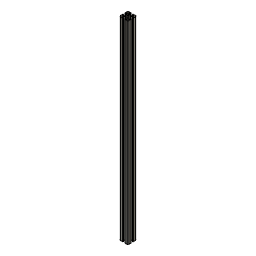
40mm X 40mm 3ft v2 (Autodesk Fusion 360 design; units mm, degrees)
Autodesk Fusion 360 part; units mm, degrees
sketch "Sketch1" plane through (0, 0, 0) normal (0, 0, 1) x (1, 0, 0)
  line L0 (4, 0) -> (14.435, 0)
  line L1 (40, 0) -> (40, 36)
  line L2 (36, 40) -> (0, 40)
  line L3 (0, 40) -> (0, 4)
  line L4 (0, 0) -> (0, 20)
  line L5 (0, 40) -> (20, 40)
  circle A0 centre (20, 20) radius 3.405
  line L6 (40, 40) -> (24.065, 40)
  line L7 (40, 40) -> (25.565, 40)
  line L8 (40, 40) -> (40, 25.565)
  line L9 (38.5, 24.065) -> (37.18, 24.065)
  line L10 (24.065, 38.5) -> (24.065, 37.18)
  line L11 (25.565, 35.68) -> (30.4344, 35.68)
  line L12 (35.68, 25.565) -> (35.68, 30.2904)
  line L13 (20, 20) -> (20, 40)
  line L14 (20, 20) -> (0, 20)
  line L15 (20, 20) -> (20, 0)
  line L16 (20, 20) -> (40, 20)
  line L17 (14.435, 35.68) -> (9.5498, 35.68)
  line L18 (15.935, 38.5) -> (15.935, 37.18)
  line L19 (4, 40) -> (14.435, 40)
  line L20 (0, 36) -> (0, 25.565)
  line L21 (1.5, 24.065) -> (2.8205, 24.065)
  line L22 (4.3205, 25.5645) -> (4.3219, 30.271)
  line L23 (25.565, 4.32) -> (1890698.4728, 3)
  line L24 (24.065, 1.5) -> (24.065, 2.82)
  line L25 (36, 0) -> (25.565, 0)
  line L26 (40, 4) -> (40, 14.435)
  line L27 (38.5, 15.935) -> (37.18, 15.935)
  line L28 (35.68, 14.435) -> (35.68, 9.7153)
  line L29 (14.435, 4.32) -> (9.7085, 4.32)
  line L30 (15.935, 1.5) -> (15.935, 2.82)
  line L31 (0, 0) -> (15.935, 0)
  line L32 (1.5, 15.935) -> (2.82, 15.935)
  line L33 (4.32, 14.435) -> (4.32, 9.5656)
  line L34 (0, 14.435) -> (0, 0)
  line L35 (0, 0) -> (15.935, 0)
  line L36 (5.9379, 30.9139) -> (12.3015, 24.1858)
  line L37 (8.8698, 34.1008) -> (15.0285, 27.5893)
  line L38 (30.9385, 5.9323) -> (24.4402, 12.1491)
  line L39 (33.9887, 8.9927) -> (27.7337, 14.9768)
  line L40 (5.903, 8.8892) -> (12.2663, 14.9767)
  line L41 (9.0615, 5.9323) -> (15.5598, 12.1491)
  line L42 (31.1111, 34.0973) -> (24.8873, 27.5855)
  line L43 (33.957, 30.8226) -> (27.7021, 24.2782)
  line L44 (27.425, 23.5872) -> (27.425, 15.6993)
  line L45 (16.2511, 12.4265) -> (23.7489, 12.4265)
  line L46 (12.575, 15.6993) -> (12.575, 23.4986)
  line L47 (15.7551, 27.2765) -> (24.1644, 27.2765)
  line L48 (35.68, 30.1316) -> (35.68, 30.2853)
  line L49 (34.0667, 30.9373) -> (34.0632, 30.9337)
  arc A1 (33.9887, 8.9927) -> (35.68, 9.7153) centre (34.68, 9.7153) ccw
  line L50 (35.68, 7.3747) -> (35.68, 9.7153)
  arc A2 (27.7021, 24.2782) -> (27.425, 23.5872) centre (28.425, 23.5872) ccw
  arc A3 (35.68, 30.2904) -> (34.0667, 30.9373) centre (34.7436, 30.2904) ccw
  arc A4 (5.9379, 30.9139) -> (4.3219, 30.271) centre (5.2579, 30.2707) ccw
  arc A5 (12.575, 23.4986) -> (12.3015, 24.1858) centre (11.575, 23.4986) ccw
  arc A6 (12.2663, 14.9767) -> (12.575, 15.6993) centre (11.575, 15.6993) ccw
  arc A7 (4.32, 9.5656) -> (5.903, 8.8892) centre (5.256, 9.5656) ccw
  arc A8 (9.0615, 5.9323) -> (9.7085, 4.32) centre (9.7085, 5.256) ccw
  arc A9 (30.2914, 4.32) -> (30.9385, 5.9323) centre (30.2914, 5.256) ccw
  arc A10 (24.4402, 12.1491) -> (23.7489, 12.4265) centre (23.7489, 11.4265) ccw
  arc A11 (16.2511, 12.4265) -> (15.5598, 12.1491) centre (16.2511, 11.4265) ccw
  arc A12 (27.425, 15.6993) -> (27.7337, 14.9768) centre (28.425, 15.6993) ccw
  arc A13 (24.1644, 27.2765) -> (24.8873, 27.5855) centre (24.1644, 28.2765) ccw
  arc A14 (15.0285, 27.5893) -> (15.7551, 27.2765) centre (15.7551, 28.2765) ccw
  arc A15 (37.18, 15.935) -> (35.68, 14.435) centre (37.18, 14.435) ccw
  arc A16 (40, 14.435) -> (38.5, 15.935) centre (38.5, 14.435) ccw
  arc A17 (35.68, 25.565) -> (37.18, 24.065) centre (37.18, 25.565) ccw
  arc A18 (38.5, 24.065) -> (40, 25.565) centre (38.5, 25.565) ccw
  arc A19 (25.565, 40) -> (24.065, 38.5) centre (25.565, 38.5) ccw
  arc A20 (24.065, 37.18) -> (25.565, 35.68) centre (25.565, 37.18) ccw
  arc A21 (14.435, 35.68) -> (15.935, 37.18) centre (14.435, 37.18) ccw
  arc A22 (15.935, 38.5) -> (14.435, 40) centre (14.435, 38.5) ccw
  arc A23 (2.8205, 24.065) -> (4.3205, 25.5645) centre (2.8205, 25.565) ccw
  arc A24 (0, 25.565) -> (1.5, 24.065) centre (1.5, 25.565) ccw
  arc A25 (4.32, 14.435) -> (2.82, 15.935) centre (2.82, 14.435) ccw
  arc A26 (1.5, 15.935) -> (0, 14.435) centre (1.5, 14.435) ccw
  arc A27 (15.935, 2.82) -> (14.435, 4.32) centre (14.435, 2.82) ccw
  arc A28 (1890698.4728, 0) -> (1890698.4728, 3) centre (1890698.4728, 1.5) ccw
  arc A29 (24.065, 1.5) -> (25.565, 0) centre (25.565, 1.5) ccw
  arc A30 (14.435, 0) -> (15.935, 1.5) centre (14.435, 1.5) ccw
  arc A31 (25.565, 4.32) -> (24.065, 2.82) centre (25.565, 2.82) ccw
  arc A32 (4, 40) -> (0, 36) centre (4, 36) ccw
  arc A33 (0, 4) -> (4, 0) centre (4, 4) ccw
  arc A34 (36, 0) -> (40, 4) centre (36, 4) ccw
  arc A35 (40, 36) -> (36, 40) centre (36, 36) ccw
  arc A36 (9.5498, 35.68) -> (8.8698, 34.1008) centre (9.5498, 34.744) ccw
  arc A37 (31.1111, 34.0973) -> (30.4344, 35.68) centre (30.4344, 34.744) ccw
  line L51 (40, 25.1972) -> (40, 36)
  line L52 (33.957, 30.8226) -> (34.0632, 30.9337)
  point P0 (20, 20)
  point P1 (40, 24.065)
  point P2 (35.68, 24.065)
  point P3 (24.065, 35.68)
  point P4 (35.68, 32.6253)
  point P5 (35.68, 7.3747)
  dimension "d1" = 40
  dimension "d2" = 40
  dimension "d8" = 15.935
  dimension "d9" = 15.935
  dimension "d10" = 4.32
  dimension "d11" = 4.32
  dimension "d16" = 90
  dimension "d17" = 90
  dimension "d22" = 4.32
  dimension "d23" = 4.32
  dimension "d24" = 4.32
  dimension "d25" = 4.32
  dimension "d26" = 8.13
  dimension "d27" = 4.32
  dimension "d28" = 14.85
  dimension "d29" = 14.85
  dimension "d30" = 7.425
  dimension "d31" = 25.2506
  dimension "d32" = 2.34
  dimension "d33" = 2.34
  dimension "d35" = 1
  dimension "d36" = 20.57
  dimension "d37" = 1
  dimension "d38" = 7.9779
  dimension "d39" = 0.9364
  dimension "d40" = 0.936
  dimension "d41" = 1
  dimension "d42" = 1
  dimension "d43" = 0.936
  dimension "d44" = 0.936
  dimension "d45" = 0.936
  dimension "d46" = 1
  dimension "d47" = 1
  dimension "d48" = 1
  dimension "d49" = 1
  dimension "d50" = 1
  dimension "d51" = 1.5
  dimension "d52" = 1.5
  dimension "d53" = 1.5
  dimension "d54" = 1.5
  dimension "d55" = 1.5
  dimension "d56" = 1.5
  dimension "d57" = 1.5
  dimension "d58" = 1.5
  dimension "d59" = 4
  dimension "d60" = 4
  dimension "d61" = 0.936
  dimension "d62" = 0.936
  constraint horizontal L0
  constraint vertical L1
  constraint horizontal L2
  constraint vertical L3
  constraint coincident L4.start L31.start
  constraint coincident P0 A0.centre
  constraint coincident L2 L6.end
  constraint perpendicular L1 L6
  constraint perpendicular L1 L7
  constraint perpendicular L7 L8
  constraint perpendicular L1 L9
  constraint perpendicular L2 L10
  constraint perpendicular L10 L11
  constraint perpendicular L9 L12
  constraint symmetric P4 L16 P5
  constraint vertical L44
  constraint horizontal L45
  constraint vertical L46
  constraint perpendicular L46 L47
  constraint parallel L12 L48
  constraint parallel L43 L49
  constraint coincident P4 L43
  constraint coincident P4 L48
  constraint coincident P5 L28
  constraint coincident P5 L39
  constraint tangent L28 A1
  constraint tangent L39 A1
  constraint coincident P5 L50.start
  constraint tangent L44 A2
  constraint tangent L43 A2
  constraint coincident P4 L49
  constraint coincident P4 L12
  constraint tangent L49 A3
  constraint tangent L12 A3
  constraint tangent L22 A4
  constraint tangent L36 A4
  constraint tangent L36 A5
  constraint tangent L46 A5
  constraint tangent L40 A6
  constraint tangent L46 A6
  constraint tangent L33 A7
  constraint tangent L40 A7
  constraint tangent L41 A8
  constraint tangent L29 A8
  constraint tangent L38 A9
  constraint tangent L23 A9
  constraint tangent L38 A10
  constraint tangent L45 A10
  constraint tangent L41 A11
  constraint tangent L45 A11
  constraint tangent L44 A12
  constraint tangent L39 A12
  constraint tangent L42 A13
  constraint tangent L47 A13
  constraint tangent L37 A14
  constraint tangent L47 A14
  constraint tangent L27 A15
  constraint tangent L28 A15
  constraint tangent L26 A16
  constraint tangent L27 A16
  constraint equal A15 A16
  constraint coincident P2 L9
  constraint coincident P2 L12
  constraint tangent L9 A17
  constraint tangent L12 A17
  constraint coincident P1 L8
  constraint coincident P1 L9
  constraint tangent L8 A18
  constraint tangent L9 A18
  constraint equal A17 A18
  constraint coincident L6.end L10
  constraint tangent L7 A19
  constraint tangent L10 A19
  constraint coincident P3 L10
  constraint coincident P3 L11
  constraint tangent L10 A20
  constraint tangent L11 A20
  constraint equal A19 A20
  constraint tangent L17 A21
  constraint tangent L18 A21
  constraint tangent L18 A22
  constraint tangent L19 A22
  constraint equal A21 A22
  constraint tangent L21 A23
  constraint tangent L22 A23
  constraint tangent L20 A24
  constraint tangent L21 A24
  constraint equal A23 A24
  constraint tangent L32 A25
  constraint tangent L33 A25
  constraint equal A23 A25
  constraint tangent L32 A26
  constraint tangent L34 A26
  constraint equal A23 A26
  constraint tangent L29 A27
  constraint tangent L30 A27
  constraint coincident L0 L15.end
  constraint coincident L1.start L0
  constraint coincident L23 A9.start
  constraint tangent L0 A28
  constraint tangent L23 A28
  constraint equal A27 A28
  constraint tangent L24 A29
  constraint tangent L25 A29
  constraint equal A27 A29
  constraint coincident L31.end L30
  constraint coincident L0 A28.start
  constraint tangent L30 A30
  constraint tangent L0 A30
  constraint tangent L23 A31
  constraint tangent L24 A31
  constraint tangent L19 A32
  constraint tangent L20 A32
  constraint coincident L3 L4.end
  constraint coincident L4.start L0
  constraint coincident L4.start L3
  constraint tangent L0 A33
  constraint tangent L3 A33
  constraint equal A32 A33
  constraint tangent L25 A34
  constraint tangent L26 A34
  constraint equal A32 A34
  constraint coincident L1 L16.end
  constraint coincident L2 L5.end
  constraint coincident L6.start L1
  constraint tangent L1 A35
  constraint tangent L2 A35
  constraint tangent L17 A36
  constraint tangent L37 A36
  constraint tangent L11 A37
  constraint tangent L42 A37
  constraint coincident L1 L51.start
  measures "d1" distance of L4.start L2.end
  measures "d2" distance of L4.start L1.start
  measures "d8" distance of L6.start L6.end
  measures "d9" distance of L6.start P1
  measures "d10" distance of P1 P2
  measures "d11" distance of L6.end P3
  measures "d16" angle of L13 L14
  measures "d17" angle of L15 L16
  measures "d22" distance of L42 L43
  measures "d23" distance of L38 L39
  measures "d24" distance of L40 L41
  measures "d25" distance of L36 L37
  measures "d26" distance of L10 L18
  measures "d27" distance of L2 L17
  measures "d28" distance of L45 L47
  measures "d29" distance of L44 L46
  measures "d30" distance of P0 L46
  measures "d31" distance of P4 P5
  measures "d32" distance of P4 L48.end
  measures "d33" distance of P4 L49.end
  measures "d35" radius of A1
  measures "d36" distance of L48.end L28.end
  measures "d37" radius of A2
  measures "d38" horizontal distance of L48.end L43.end
  measures "d39" radius of A3
  measures "d40" radius of A4
  measures "d41" radius of A5
  measures "d42" radius of A6
  measures "d43" radius of A7
  measures "d44" radius of A8
  measures "d45" radius of A9
  measures "d46" radius of A10
  measures "d47" radius of A11
  measures "d48" radius of A12
  measures "d49" radius of A13
  measures "d50" radius of A14
  measures "d51" radius of A15
  measures "d52" radius of A17
  measures "d53" radius of A19
  measures "d54" radius of A21
  measures "d55" radius of A23
  measures "d56" radius of A27
  measures "d57" radius of A30
  measures "d58" radius of A31
  measures "d59" radius of A32
  measures "d60" radius of A35
  measures "d61" radius of A36
  measures "d62" radius of A37
extrude "Extrude1" add sketch "Sketch1" along normal blind 914.4 contours L0 L3 L4 A0 L14 L15 L29 L30 L31 L32 L33 L34 L35 L40 L41 L45 L46 A6 A7 A8 A11 A25 A26 A27 A30 A33 | L2 L3 L5 A0 L13 L14 L17 L18 L19 L20 L21 L22 L36 L37 L46 L47 A4 A5 A14 A21 A22 A23 A24 A32 A36 | L1 L2 A0 L6 L7 L8 L9 L10 L11 L12 L13 L16 L42 L43 L44 L47 L48 L49 A2 A3 A13 A17 A18 A19 A20 A35 A37 L51 L52 | L1 A0 L15 L16 L23 L26 L27 L28 L38 L39 L44 L45 A1 A9 A10 A12 A15 A16 | L1 L23 L24 L25 L26 A29 A31 A34
